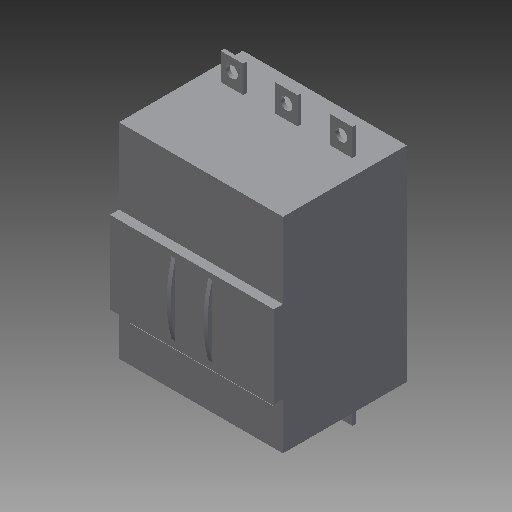
# Autodesk Inventor part: nzm1_3p_p1
Saved by Autodesk Inventor 2019.3 (Build 233278000, 278)
## iProperties
Category: PARTsolutions
Company: MOELLER
Created: 2018-10-25
Part Number: nzm1_3p_p1
Material: Generic
Catalog Web Link: www.cadenas.de
Description: Leistungsschalter 3p_p1-Leistungsschalter 3p
Vendor: MOELLER
Document SubType Name: Modeling
Designer: psadmin
Manufacturer: MOELLER
Mass: 710.16 g
Surface Area: 522.631 cm^2
Volume: 710.16 cm^3
Density: 1 g/cm^3
Appearance: PSOLRGB-192-192-192
PSOL_IDENT_0: {$CADENAS_DATA\23d-libs\moeller\circuit_breaker\parts\nzm1_3p_p1.prj},178 {VTYP=3D},{NB=nzm1_3p_p1},
PSOL_IDENT_1: {LINA=nzm1_3p_p1},{NN=Leistungsschalter 3p_p1},{DATE=05.10.2018 14:14:19},{GEOMDATE=14.05.2018 10:43
PSOL_IDENT_2: :05},{VERSION=},{LINEID=310},{WBVAR=},{WBNUMERIC=}  {NB=nzm1_3p_p1},{LINA=nzm1_3p_p1},{KT=DUMMY},{BM
PSOL_IDENT_3: ENB=nzm1_3p_p1},{EPLAN=}
NN: Leistungsschalter 3p_p1
NT: Leistungsschalter 3p
NB: nzm1_3p_p1
NBSYN: $BMENB.
LINA: nzm1_3p_p1
BMENB: nzm1_3p_p1
SUPPLIER: MOELLER
ARTICLENO: nzm1_3p_p1
BOMINFO: nzm1_3p_p1
CREATOR: CADENAS GmbH
Title: nzm1_3p_p1
Author: Cadenas PARTsolutions
Comments: Leistungsschalter 3p
Autodesk Inventor part; units mm, degrees
sketch "Sketch_1" plane through (0, 0, 0) normal (1, 0, 0) x (0, 1, 0)
  line L0 (-30.3, 73) -> (-30.3, 68)
  line L1 (-30.3, 68) -> (-56.2, 68)
  line L2 (-56.2, 68) -> (-56.2, 0)
  line L3 (-56.2, 0) -> (56.2, 0)
  line L4 (56.2, 0) -> (56.2, 68)
  line L5 (56.2, 68) -> (14.7, 68)
  line L6 (14.7, 68) -> (14.7, 73)
  line L7 (14.7, 73) -> (-30.3, 73)
  constraints: 16 end point
extrude "Extrusion1" add sketch "Sketch_1" along normal blind 90
sketch "Sketch_3" plane through (45, 0, 0) normal (1, 0, 0) x (0, 0, -1)
  line L0 (-69, -56.2) -> (-65.75, -56.2)
  line L1 (-65.75, -56.2) -> (-66, -55.95)
  line L2 (-66, -55.95) -> (-66, -36.15)
  line L3 (-66, -36.15) -> (-69, -36.15)
  line L4 (-69, -36.15) -> (-69, -56.2)
  constraints: 10 end point
extrude "Extrusion2" cut sketch "Sketch_3" along normal mid plane 79.1
sketch "Sketch_2" plane through (45, 0, 0) normal (1, 0, 0) x (0, 0, -1)
  line L0 (-68.007, -56.2) -> (-66, -56.2)
  line L1 (-66, -56.2) -> (-66, -36.4)
  line L2 (-66, -36.4) -> (-68.007, -36.4)
  line L3 (-68.007, -36.4) -> (-68.007, -56.2)
  constraints: 8 end point
extrude "Extrusion3" add sketch "Sketch_2" along normal mid plane 78.6
sketch "Sketch_4" plane through (35.991, 0, 0) normal (1, 0, 0) x (0, 0, -1)
  arc A0 (-73, 11.7765) -> (-73, -27.3765) centre (-0.6, -7.8) ccw
  line L0 (-73, -27.3765) -> (-73, 11.7765)
  constraints: 2 end point, 2 point on circle, 1 centre point
extrude "Extrusion4" add sketch "Sketch_4" against normal blind 2.182
sketch "Sketch_5" plane through (54.009, 0, 0) normal (1, 0, 0) x (0, 0, -1)
  arc A0 (-73, 11.7765) -> (-73, -27.3765) centre (-0.6, -7.8) ccw
  line L0 (-73, -27.3765) -> (-73, 11.7765)
  constraints: 2 end point, 2 point on circle, 1 centre point
extrude "Extrusion5" add sketch "Sketch_5" along normal blind 2.182
sketch "Sketch_7" plane through (0, 0, 21) normal (0, 0, 1) x (1, 0, 0)
  line L0 (8.9, -71.05) -> (21.1, -71.05)
  line L1 (21.1, -71.05) -> (21.1, -54.2)
  line L2 (21.1, -54.2) -> (38.9, -54.2)
  line L3 (38.9, -54.2) -> (38.9, -71.05)
  line L4 (38.9, -71.05) -> (51.1, -71.05)
  line L5 (51.1, -71.05) -> (51.1, -54.2)
  line L6 (51.1, -54.2) -> (68.9, -54.2)
  line L7 (68.9, -54.2) -> (68.9, -71.05)
  line L8 (68.9, -71.05) -> (81.1, -71.05)
  line L9 (81.1, -71.05) -> (81.1, 71.05)
  line L10 (81.1, 71.05) -> (68.9, 71.05)
  line L11 (68.9, 71.05) -> (68.9, 54.2)
  line L12 (68.9, 54.2) -> (51.1, 54.2)
  line L13 (51.1, 54.2) -> (51.1, 71.05)
  line L14 (51.1, 71.05) -> (38.9, 71.05)
  line L15 (38.9, 71.05) -> (38.9, 54.2)
  line L16 (38.9, 54.2) -> (21.1, 54.2)
  line L17 (21.1, 54.2) -> (21.1, 71.05)
  line L18 (21.1, 71.05) -> (8.9, 71.05)
  line L19 (8.9, 71.05) -> (8.9, -71.05)
  circle A0 centre (75, 64.05) radius 3.25
  circle A1 centre (75, -64.05) radius 3.25
  circle A2 centre (45, 64.05) radius 3.25
  circle A3 centre (45, -64.05) radius 3.25
  circle A4 centre (15, 64.05) radius 3.25
  circle A5 centre (15, -64.05) radius 3.25
  constraints: 40 end point, 6 centre point
extrude "Extrusion6" add sketch "Sketch_7" against normal blind 2
ref_plane "FOR_P2_XY" through (0, 56.2, 0) normal (0, 1, 0) x (1, 0, 0)
ref_plane "FOR_P2_YZ" through (0, 56.2, 0) normal (1, 0, 0) x (0, 0, -1)
ref_plane "FOR_P2_ZX" through (0, 56.2, 0) normal (0, 0, -1) x (0, 1, 0)
ref_plane "FOR_P22_XY" through (90, -56.2, 0) normal (0, -1, 0) x (1, 0, 0)
ref_plane "FOR_P22_YZ" through (90, -56.2, 0) normal (1, 0, 0) x (0, 0, 1)
ref_plane "FOR_P22_ZX" through (90, -56.2, 0) normal (0, 0, 1) x (0, -1, 0)
ref_plane "P1_XY" through (0, 0, 0) normal (0, 0, 1) x (1, 0, 0)
ref_plane "P1_YZ" through (0, 0, 0) normal (1, 0, 0) x (0, 1, 0)
ref_plane "P1_ZX" through (0, 0, 0) normal (0, 1, 0) x (0, 0, 1)
ref_plane "P3_XY" through (45, -5.518, 73) normal (0, 0, 1) x (1, 0, 0)
ref_plane "P3_YZ" through (45, -5.518, 73) normal (1, 0, 0) x (0, 1, 0)
ref_plane "P3_ZX" through (45, -5.518, 73) normal (0, 1, 0) x (0, 0, 1)
body "Solid1"
